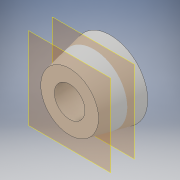
# Autodesk Inventor part: Patas
Saved by Autodesk Inventor 2019.4 (Build 234330000, 330)
## iProperties
Created: 2019-07-30
Part Number: Patas
Material: Genérico
Document SubType Name: Modeling
Designer: Irene
Density: 1 g/cm^3
Appearance: Valor por defecto
Author: Irene
Autodesk Inventor part; units mm, degrees
ref_plane "YZ Plane" through (0, 0, 0) normal (1, 0, 0) x (0, 1, 0)
ref_plane "XZ Plane" through (0, 0, 0) normal (0, 1, 0) x (-1, 0, 0)
sketch "Boceto1" plane through (0, 0, 0) normal (0, 0, 1) x (1, 0, 0)
  circle A0 centre (0, 0) radius 11
  dimension "d0" = 22
  constraints: 1 centre point, 1 coincident
  measures "d0" diameter of A0
ref_plane "Plano de trabajo3" through (0, 0, 5) normal (0, 0, 1) x (1, 0, 0)
sketch "Boceto3" plane through (0, 0, 5) normal (0, 0, 1) x (1, 0, 0)
  circle A0 centre (0, 0) radius 4.5
  circle A1 centre (0, 0) radius 1.5
  dimension "d5" = 9
  dimension "d6" = 3
  constraints: 2 centre point, 2 coincident
  measures "d5" diameter of A0
  measures "d6" diameter of A1
ref_plane "Plano de trabajo4" through (0, 0, 12) normal (0, 0, 1) x (1, 0, 0)
sketch "Boceto4" plane through (0, 0, 12) normal (0, 0, 1) x (1, 0, 0)
  circle A0 centre (0, 0) radius 8.5
  dimension "d8" = 17
  constraints: 1 centre point, 1 coincident
  measures "d8" diameter of A0
loft "Solevación1" add profiles "Boceto1", "Boceto4"
hole "Agujero3" at (0, 0, 5) direction (0, 0, 1) diameter 9 depth 7
sketch "Boceto5" plane through (0, 0, 5) normal (0, 0, 1) x (1, 0, 0)
  point P0 (0, 0)
  point P1 (0.0057, -0.0188)
hole "Agujero4" at (0.0057, -0.0188, 5) direction (0, 0, -1) diameter 3.2 end through all
